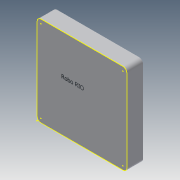
# Autodesk Inventor part: robo rio
Saved by Autodesk Inventor 2014 (Build 180170000, 170)
## iProperties
Created: 2016-01-12
Part Number: robo rio
Material: Generic
Document SubType Name: Modeling
Designer: Paul
Density: 1 g/cm^3
Appearance: Default
Author: Paul
Autodesk Inventor part; units mm, degrees
ref_plane "YZ Plane" through (0, 0, 0) normal (1, 0, 0) x (0, 1, 0)
ref_plane "XZ Plane" through (0, 0, 0) normal (0, 1, 0) x (-1, 0, 0)
ref_plane "XY Plane" through (0, 0, 0) normal (0, 0, 1) x (1, 0, 0)
sketch "Sketch1" plane through (0, 0, 0) normal (0, 0, 1) x (1, 0, 0)
  line L0 (6.35, 0) -> (136.525, 0)
  line L1 (142.875, 6.35) -> (142.875, 136.525)
  line L2 (136.525, 142.875) -> (6.35, 142.875)
  line L3 (0, 136.525) -> (0, 6.35)
  arc A0 (6.35, 142.875) -> (0, 136.525) centre (6.35, 136.525) ccw
  arc A1 (142.875, 136.525) -> (136.525, 142.875) centre (136.525, 136.525) ccw
  arc A2 (136.525, 0) -> (142.875, 6.35) centre (136.525, 6.35) ccw
  arc A3 (0, 6.35) -> (6.35, 0) centre (6.35, 6.35) ccw
  point P0 (0, 0)
  point P1 (142.875, 142.875)
  point P2 (142.875, 0)
  point P3 (0, 142.875)
  dimension "d0" = 142.875
  dimension "d1" = 142.875
  dimension "d2" = 6.35
  constraints: 8 end point, 8 point on circle, 8 point on line, 8 tangent, 4 centre point, 3 equal radius, 2 parallel, 1 horizontal, 1 perpendicular
  measures "d0" distance of point (0, 142.875) point (142.875, 142.875)
  measures "d1" distance of point (142.875, 142.875) point (142.875, 0)
  measures "d2" radius of A0
extrude "Extrusion1" add sketch "Sketch1" along normal blind 25.4
sketch "Sketch2" plane through (0, 0, 25.4) normal (0, 0, 1) x (1, 0, 0)
  line L0 (136.525, 142.875) -> (6.35, 142.875) projected
  arc A0 (6.35, 142.875) -> (0, 136.525) centre (6.35, 136.525) ccw projected
  line L1 (0, 136.525) -> (0, 6.35) projected
  arc A1 (0, 6.35) -> (6.35, 0) centre (6.35, 6.35) ccw projected
  line L2 (6.35, 0) -> (136.525, 0) projected
  arc A2 (136.525, 0) -> (142.875, 6.35) centre (136.525, 6.35) ccw projected
  line L3 (142.875, 6.35) -> (142.875, 136.525) projected
  arc A3 (142.875, 136.525) -> (136.525, 142.875) centre (136.525, 136.525) ccw projected
  line L4 (38.5402, 84.1852) -> (110.9143, 84.1852) construction
  line L5 (110.9143, 84.1852) -> (110.9143, 57.8674) construction
  line L6 (110.9143, 57.8674) -> (38.5402, 57.8674) construction
  line L7 (38.5402, 57.8674) -> (38.5402, 84.1852) construction
  point P0 (0, 0)
  constraints: 2 other
body "Solid1"
